TOILETS TEXT (Autodesk Fusion 360 design; units mm, degrees)
Autodesk Fusion 360 part; units mm, degrees
note: some values were not read from the file. Chosen so that the rebuilt part matches the saved one: which bodies a step acts on; the layout of a text.
sketch "Sketch1" plane through (0, 0, 0) normal (0, 1, 0) x (1, 0, 0)
  line L0 (-70, -1) -> (-23.1738, -1) construction
  line L1 (-23.1738, -1) -> (-23.1738, 9) construction
  line L2 (-23.1738, 9) -> (-70, 9) construction
  line L3 (-70, 9) -> (-70, -1) construction
  text T0 "TOILETS" font "Arial Black" height 10 bold align ink ink in box 0 x 0 at (-69.99, -0.98) x (1, 0) y (0, 1) spacing 1 kerned height is em
  constraint perpendicular L0 L1
  constraint parallel L0 L2
  constraint parallel L1 L3
extrude "Extrude1" add sketch "Sketch1" along normal blind 5 text T0 makes body 1 at (-62.1154, 0, -3.1409) makes body 2 at (-25.1005, 0, -2.8954) makes body 3 at (-43.7205, 1.6667, -1.5281) makes body 4 at (-34.7556, 1.6667, -6.3003) makes body 5 at (-50.3855, 1.6667, -1.5281) makes body 6 at (-51.9724, 1.6667, -3.9142) makes body 7 at (-67.7488, 1.6667, -6.3003)
sketch "Sketch2" plane through (0, 0, 0) normal (0, 1, 0) x (1, 0, 0)
  line L0 (-20.1638, -3.98) -> (-72.99, -3.98)
  line L1 (-72.99, -3.98) -> (-72.99, 9.3003)
  line L2 (-72.99, 9.3003) -> (-20.1638, 9.3003)
  line L3 (-20.1638, 9.3003) -> (-20.1638, -3.98)
  point P0 (-69.99, 6.3003)
extrude "Extrude2" add sketch "Sketch2" along normal blind 2 bodies 1 2 3 4 5 6 7
